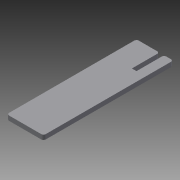
# Autodesk Inventor part: pa28-bellcrank-rigging-tool
Saved by Autodesk Inventor 2015 (Build 190159000, 159)
## iProperties
Created: 2016-01-21
Part Number: pa28-bellcrank-rigging-tool
Material: Generic
Document SubType Name: Modeling
Designer: bovine
Density: 1 g/cm^3
Appearance: Default
Author: bovine
Autodesk Inventor part; units mm, degrees
ref_plane "YZ Plane" through (0, 0, 0) normal (1, 0, 0) x (0, 1, 0)
ref_plane "XZ Plane" through (0, 0, 0) normal (0, 1, 0) x (-1, 0, 0)
ref_plane "XY Plane" through (0, 0, 0) normal (0, 0, 1) x (1, 0, 0)
sketch "Sketch1" plane through (0, 0, 0) normal (0, 1, 0) x (-1, 0, 0)
  line L0 (25.4, 89.6874) -> (0, 89.6874)
  line L1 (0, 89.6874) -> (0, 0)
  line L2 (0, 0) -> (6.35, 0)
  line L3 (25.4, 0) -> (25.4, 89.6874)
  line L4 (9.525, 0) -> (9.525, 19.05)
  line L5 (9.525, 19.05) -> (6.35, 19.05)
  line L6 (6.35, 19.05) -> (6.35, 0)
  line L7 (9.525, 0) -> (25.4, 0)
  dimension "d0" = 25.4
  dimension "d1" = 89.6874
  dimension "d2" = 3.175
  dimension "d3" = 19.05
  constraints: 16 end point, 4 parallel, 1 coincident, 1 horizontal, 1 perpendicular
  measures "d0" distance of L3.start L1.end
  measures "d1" distance of L1.end L0.end
  measures "d2" distance of L5.end L4.end
  measures "d3" distance of L4.end L4.start
extrude "Extrusion1" add sketch "Sketch1" along normal blind 3.175
fillet "Fillet1" radius 1.5748 6 edges at (0, 1.5875, 0) (-25.4, 1.5875, 0) (-6.35, 1.5875, 0) (-9.525, 1.5875, 0) (-25.4, 1.5875, 89.6874) (0, 1.5875, 89.6874)
sketch "Sketch2" plane through (0, 0, 0) normal (0, -1, 0) x (1, 0, 0)
  line L0 (-20.5155, 21.5283) -> (-20.5155, 87.253) construction
  line L1 (-20.5155, 87.253) -> (-16.4672, 87.253) construction
  line L2 (-16.4672, 87.253) -> (-16.4672, 21.5283) construction
  line L3 (-16.4672, 21.5283) -> (-20.5155, 21.5283) construction
  spline S0 degree 2 poles (-19.4608, 23.7637) (-19.2632, 23.7637) (-18.9076, 23.6229) (-18.7841, 23.4969) knots 0 0 0 1 2 2 2
  spline S1 degree 2 poles (-18.7841, 23.4969) (-18.6284, 23.3388) (-18.4679, 22.9115) (-18.4679, 22.5855) knots 0 0 0 1 2 2 2
  line L4 (-18.4679, 22.5855) -> (-18.4679, 22.2422)
  line L5 (-18.4679, 22.2422) -> (-17.3317, 22.2422)
  line L6 (-17.3317, 22.2422) -> (-17.3317, 21.8371)
  line L7 (-17.3317, 21.8371) -> (-20.3797, 21.8371)
  line L8 (-20.3797, 21.8371) -> (-20.3797, 22.6028)
  spline S2 degree 2 poles (-20.3797, 22.6028) (-20.3797, 22.8745) (-20.2908, 23.2549) (-20.1895, 23.4006) knots 0 0 0 1 2 2 2
  spline S3 degree 2 poles (-20.1895, 23.4006) (-20.0734, 23.571) (-19.7152, 23.7637) (-19.4608, 23.7637) knots 0 0 0 1 2 2 2
  spline S4 degree 2 poles (-19.4485, 23.3413) (-19.6066, 23.3413) (-19.8387, 23.2326) (-19.9129, 23.1215) knots 0 0 0 1 2 2 2
  spline S5 degree 2 poles (-19.9129, 23.1215) (-19.9771, 23.0252) (-20.0289, 22.7683) (-20.0289, 22.5781) knots 0 0 0 1 2 2 2
  line L9 (-20.0289, 22.5781) -> (-20.0289, 22.2422)
  line L10 (-20.0289, 22.2422) -> (-18.8137, 22.2422)
  line L11 (-18.8137, 22.2422) -> (-18.8137, 22.5188)
  spline S6 degree 2 poles (-18.8137, 22.5188) (-18.8137, 22.7658) (-18.8927, 23.0696) (-18.9965, 23.1684) knots 0 0 0 1 2 2 2
  spline S7 degree 2 poles (-18.9965, 23.1684) (-19.0879, 23.2598) (-19.3028, 23.3413) (-19.4485, 23.3413) knots 0 0 0 1 2 2 2
  line L12 (-17.3317, 24.5121) -> (-17.3317, 24.1268)
  line L13 (-17.3317, 24.1268) -> (-19.6189, 24.1268)
  line L14 (-19.6189, 24.1268) -> (-19.6189, 24.5121)
  line L15 (-19.6189, 24.5121) -> (-17.3317, 24.5121)
  line L16 (-19.9993, 24.5393) -> (-19.9993, 24.1021)
  line L17 (-19.9993, 24.1021) -> (-20.3994, 24.1021)
  line L18 (-20.3994, 24.1021) -> (-20.3994, 24.5393)
  line L19 (-20.3994, 24.5393) -> (-19.9993, 24.5393)
  spline S8 degree 2 poles (-18.5371, 26.9945) (-17.964, 26.9945) (-17.2872, 26.4486) (-17.2872, 26.0312) knots 0 0 0 1 2 2 2
  spline S9 degree 2 poles (-17.2872, 26.0312) (-17.2872, 25.8607) (-17.3663, 25.5989) (-17.4478, 25.4631) knots 0 0 0 1 2 2 2
  line L20 (-17.4478, 25.4631) -> (-16.4894, 25.4631)
  line L21 (-16.4894, 25.4631) -> (-16.4894, 25.0777)
  line L22 (-16.4894, 25.0777) -> (-19.6189, 25.0777)
  line L23 (-19.6189, 25.0777) -> (-19.6189, 25.4631)
  line L24 (-19.6189, 25.4631) -> (-19.3793, 25.4631)
  spline S10 degree 2 poles (-19.3793, 25.4631) (-19.5102, 25.6063) (-19.6831, 25.9571) (-19.6831, 26.1621) knots 0 0 0 1 2 2 2
  spline S11 degree 2 poles (-19.6831, 26.1621) (-19.6831, 26.5548) (-19.0607, 26.9945) (-18.5371, 26.9945) knots 0 0 0 1 2 2 2
  spline S12 degree 2 poles (-18.4926, 26.5968) (-18.8853, 26.5968) (-19.3176, 26.3473) (-19.3176, 26.0682) knots 0 0 0 1 2 2 2
  spline S13 degree 2 poles (-19.3176, 26.0682) (-19.3176, 25.9052) (-19.1718, 25.5989) (-19.0582, 25.4631) knots 0 0 0 1 2 2 2
  line L25 (-19.0582, 25.4631) -> (-17.759, 25.4631)
  spline S14 degree 2 poles (-17.759, 25.4631) (-17.6874, 25.6137) (-17.633, 25.8286) (-17.633, 25.9669) knots 0 0 0 1 2 2 2
  spline S15 degree 2 poles (-17.633, 25.9669) (-17.633, 26.2658) (-18.0727, 26.5968) (-18.4926, 26.5968) knots 0 0 0 1 2 2 2
  spline S16 degree 2 poles (-17.2798, 28.3876) (-17.2798, 27.8392) (-17.8948, 27.2365) (-18.463, 27.2365) knots 0 0 0 1 2 2 2
  spline S17 degree 2 poles (-18.463, 27.2365) (-19.0212, 27.2365) (-19.6831, 27.8219) (-19.6831, 28.2937) knots 0 0 0 1 2 2 2
  spline S18 degree 2 poles (-19.6831, 28.2937) (-19.6831, 28.5061) (-19.5596, 28.8346) (-19.4287, 28.9557) knots 0 0 0 1 2 2 2
  spline S19 degree 2 poles (-19.4287, 28.9557) (-19.2978, 29.0792) (-18.9199, 29.2101) (-18.6457, 29.2101) knots 0 0 0 1 2 2 2
  line L26 (-18.6457, 29.2101) -> (-18.4358, 29.2101)
  line L27 (-18.4358, 29.2101) -> (-18.4358, 27.6268)
  spline S20 degree 2 poles (-18.4358, 27.6268) (-18.0381, 27.6268) (-17.6157, 28.0269) (-17.6157, 28.3826) knots 0 0 0 1 2 2 2
  spline S21 degree 2 poles (-17.6157, 28.3826) (-17.6157, 28.5086) (-17.6725, 28.7531) (-17.717, 28.8519) knots 0 0 0 1 2 2 2
  spline S22 degree 2 poles (-17.717, 28.8519) (-17.7664, 28.9557) (-17.8529, 29.0989) (-17.8924, 29.1459) knots 0 0 0 1 2 2 2
  line L28 (-17.8924, 29.1459) -> (-17.8924, 29.1681)
  line L29 (-17.8924, 29.1681) -> (-17.4725, 29.1681)
  spline S23 degree 2 poles (-17.4725, 29.1681) (-17.4453, 29.1014) (-17.3663, 28.8989) (-17.344, 28.8198) knots 0 0 0 1 2 2 2
  spline S24 degree 2 poles (-17.344, 28.8198) (-17.3119, 28.7087) (-17.2798, 28.5259) (-17.2798, 28.3876) knots 0 0 0 1 2 2 2
  spline S25 degree 2 poles (-18.7297, 28.8346) (-18.8853, 28.8297) (-19.1126, 28.7655) (-19.1891, 28.7037) knots 0 0 0 1 2 2 2
  spline S26 degree 2 poles (-19.1891, 28.7037) (-19.2756, 28.637) (-19.367, 28.4271) (-19.367, 28.2715) knots 0 0 0 1 2 2 2
  spline S27 degree 2 poles (-19.367, 28.2715) (-19.367, 28.1183) (-19.2756, 27.9034) (-19.1867, 27.8145) knots 0 0 0 1 2 2 2
  spline S28 degree 2 poles (-19.1867, 27.8145) (-19.0953, 27.7281) (-18.8754, 27.6391) (-18.7297, 27.6268) knots 0 0 0 1 2 2 2
  line L30 (-18.7297, 27.6268) -> (-18.7297, 28.8346)
  line L31 (-19.2064, 30.8131) -> (-19.2064, 30.7934)
  spline S29 degree 2 poles (-19.2064, 30.7934) (-19.2188, 30.7489) (-19.2237, 30.6526) (-19.2237, 30.5859) knots 0 0 0 1 2 2 2
  spline S30 degree 2 poles (-19.2237, 30.5859) (-19.2237, 30.4303) (-19.0879, 30.124) (-18.9545, 29.9857) knots 0 0 0 1 2 2 2
  line L32 (-18.9545, 29.9857) -> (-17.3317, 29.9857)
  line L33 (-17.3317, 29.9857) -> (-17.3317, 29.6003)
  line L34 (-17.3317, 29.6003) -> (-19.6189, 29.6003)
  line L35 (-19.6189, 29.6003) -> (-19.6189, 29.9857)
  line L36 (-19.6189, 29.9857) -> (-19.2781, 29.9857)
  spline S31 degree 2 poles (-19.2781, 29.9857) (-19.4658, 30.1956) (-19.6189, 30.5093) (-19.6189, 30.6575) knots 0 0 0 1 2 2 2
  spline S32 degree 2 poles (-19.6189, 30.6575) (-19.6189, 30.7168) (-19.614, 30.7761) (-19.6066, 30.8131) knots 0 0 0 1 2 2 2
  line L37 (-19.6066, 30.8131) -> (-19.2064, 30.8131)
  line L38 (-17.3317, 32.1222) -> (-20.3797, 33.1497)
  line L39 (-20.3797, 33.1497) -> (-20.3797, 33.6487)
  line L40 (-20.3797, 33.6487) -> (-17.3317, 34.6762)
  line L41 (-17.3317, 34.6762) -> (-17.3317, 34.2489)
  line L42 (-17.3317, 34.2489) -> (-18.1838, 33.9723)
  line L43 (-18.1838, 33.9723) -> (-18.1838, 32.8089)
  line L44 (-18.1838, 32.8089) -> (-17.3317, 32.5322)
  line L45 (-17.3317, 32.5322) -> (-17.3317, 32.1222)
  line L46 (-18.5296, 33.8611) -> (-19.9647, 33.3893)
  line L47 (-19.9647, 33.3893) -> (-18.5296, 32.92)
  line L48 (-18.5296, 32.92) -> (-18.5296, 33.8611)
  line L49 (-17.3317, 35.3283) -> (-17.3317, 34.943)
  line L50 (-17.3317, 34.943) -> (-19.6189, 34.943)
  line L51 (-19.6189, 34.943) -> (-19.6189, 35.3283)
  line L52 (-19.6189, 35.3283) -> (-17.3317, 35.3283)
  line L53 (-19.9993, 35.3555) -> (-19.9993, 34.9183)
  line L54 (-19.9993, 34.9183) -> (-20.3994, 34.9183)
  line L55 (-20.3994, 34.9183) -> (-20.3994, 35.3555)
  line L56 (-20.3994, 35.3555) -> (-19.9993, 35.3555)
  line L57 (-17.3317, 36.2867) -> (-17.3317, 35.9013)
  line L58 (-17.3317, 35.9013) -> (-20.5155, 35.9013)
  line L59 (-20.5155, 35.9013) -> (-20.5155, 36.2867)
  line L60 (-20.5155, 36.2867) -> (-17.3317, 36.2867)
  spline S33 degree 2 poles (-17.2798, 37.8452) (-17.2798, 37.2969) (-17.8948, 36.6942) (-18.463, 36.6942) knots 0 0 0 1 2 2 2
  spline S34 degree 2 poles (-18.463, 36.6942) (-19.0212, 36.6942) (-19.6831, 37.2796) (-19.6831, 37.7514) knots 0 0 0 1 2 2 2
  spline S35 degree 2 poles (-19.6831, 37.7514) (-19.6831, 37.9638) (-19.5596, 38.2923) (-19.4287, 38.4134) knots 0 0 0 1 2 2 2
  spline S36 degree 2 poles (-19.4287, 38.4134) (-19.2978, 38.5369) (-18.9199, 38.6678) (-18.6457, 38.6678) knots 0 0 0 1 2 2 2
  line L61 (-18.6457, 38.6678) -> (-18.4358, 38.6678)
  line L62 (-18.4358, 38.6678) -> (-18.4358, 37.0845)
  spline S37 degree 2 poles (-18.4358, 37.0845) (-18.0381, 37.0845) (-17.6157, 37.4846) (-17.6157, 37.8403) knots 0 0 0 1 2 2 2
  spline S38 degree 2 poles (-17.6157, 37.8403) (-17.6157, 37.9663) (-17.6725, 38.2108) (-17.717, 38.3096) knots 0 0 0 1 2 2 2
  spline S39 degree 2 poles (-17.717, 38.3096) (-17.7664, 38.4134) (-17.8529, 38.5566) (-17.8924, 38.6035) knots 0 0 0 1 2 2 2
  line L63 (-17.8924, 38.6035) -> (-17.8924, 38.6258)
  line L64 (-17.8924, 38.6258) -> (-17.4725, 38.6258)
  spline S40 degree 2 poles (-17.4725, 38.6258) (-17.4453, 38.5591) (-17.3663, 38.3565) (-17.344, 38.2775) knots 0 0 0 1 2 2 2
  spline S41 degree 2 poles (-17.344, 38.2775) (-17.3119, 38.1664) (-17.2798, 37.9836) (-17.2798, 37.8452) knots 0 0 0 1 2 2 2
  spline S42 degree 2 poles (-18.7297, 38.2923) (-18.8853, 38.2874) (-19.1126, 38.2232) (-19.1891, 38.1614) knots 0 0 0 1 2 2 2
  spline S43 degree 2 poles (-19.1891, 38.1614) (-19.2756, 38.0947) (-19.367, 37.8848) (-19.367, 37.7292) knots 0 0 0 1 2 2 2
  spline S44 degree 2 poles (-19.367, 37.7292) (-19.367, 37.576) (-19.2756, 37.3611) (-19.1867, 37.2722) knots 0 0 0 1 2 2 2
  spline S45 degree 2 poles (-19.1867, 37.2722) (-19.0953, 37.1858) (-18.8754, 37.0968) (-18.7297, 37.0845) knots 0 0 0 1 2 2 2
  line L65 (-18.7297, 37.0845) -> (-18.7297, 38.2923)
  line L66 (-19.2064, 40.2708) -> (-19.2064, 40.251)
  spline S46 degree 2 poles (-19.2064, 40.251) (-19.2188, 40.2066) (-19.2237, 40.1103) (-19.2237, 40.0436) knots 0 0 0 1 2 2 2
  spline S47 degree 2 poles (-19.2237, 40.0436) (-19.2237, 39.888) (-19.0879, 39.5817) (-18.9545, 39.4433) knots 0 0 0 1 2 2 2
  line L67 (-18.9545, 39.4433) -> (-17.3317, 39.4433)
  line L68 (-17.3317, 39.4433) -> (-17.3317, 39.058)
  line L69 (-17.3317, 39.058) -> (-19.6189, 39.058)
  line L70 (-19.6189, 39.058) -> (-19.6189, 39.4433)
  line L71 (-19.6189, 39.4433) -> (-19.2781, 39.4433)
  spline S48 degree 2 poles (-19.2781, 39.4433) (-19.4658, 39.6533) (-19.6189, 39.967) (-19.6189, 40.1152) knots 0 0 0 1 2 2 2
  spline S49 degree 2 poles (-19.6189, 40.1152) (-19.6189, 40.1745) (-19.614, 40.2338) (-19.6066, 40.2708) knots 0 0 0 1 2 2 2
  line L72 (-19.6066, 40.2708) -> (-19.2064, 40.2708)
  spline S50 degree 2 poles (-18.4753, 42.4494) (-17.8973, 42.4494) (-17.2675, 41.8936) (-17.2675, 41.4292) knots 0 0 0 1 2 2 2
  spline S51 degree 2 poles (-17.2675, 41.4292) (-17.2675, 40.9525) (-17.9171, 40.4067) (-18.4753, 40.4067) knots 0 0 0 1 2 2 2
  spline S52 degree 2 poles (-18.4753, 40.4067) (-19.0483, 40.4067) (-19.6831, 40.9698) (-19.6831, 41.4292) knots 0 0 0 1 2 2 2
  spline S53 degree 2 poles (-19.6831, 41.4292) (-19.6831, 41.8936) (-19.0508, 42.4494) (-18.4753, 42.4494) knots 0 0 0 1 2 2 2
  spline S54 degree 2 poles (-18.4753, 42.0517) (-18.9199, 42.0517) (-19.3522, 41.7281) (-19.3522, 41.4292) knots 0 0 0 1 2 2 2
  spline S55 degree 2 poles (-19.3522, 41.4292) (-19.3522, 41.1304) (-18.9199, 40.8043) (-18.4753, 40.8043) knots 0 0 0 1 2 2 2
  spline S56 degree 2 poles (-18.4753, 40.8043) (-18.043, 40.8043) (-17.5984, 41.1304) (-17.5984, 41.4292) knots 0 0 0 1 2 2 2
  spline S57 degree 2 poles (-17.5984, 41.4292) (-17.5984, 41.7256) (-18.0356, 42.0517) (-18.4753, 42.0517) knots 0 0 0 1 2 2 2
  line L73 (-17.3317, 44.6403) -> (-17.3317, 44.2549)
  line L74 (-17.3317, 44.2549) -> (-18.6359, 44.2549)
  spline S58 degree 2 poles (-18.6359, 44.2549) (-18.7939, 44.2549) (-19.0656, 44.2253) (-19.1471, 44.1808) knots 0 0 0 1 2 2 2
  spline S59 degree 2 poles (-19.1471, 44.1808) (-19.2336, 44.1339) (-19.3176, 43.9659) (-19.3176, 43.8227) knots 0 0 0 1 2 2 2
  spline S60 degree 2 poles (-19.3176, 43.8227) (-19.3176, 43.6794) (-19.1644, 43.3756) (-19.0409, 43.2299) knots 0 0 0 1 2 2 2
  line L75 (-19.0409, 43.2299) -> (-17.3317, 43.2299)
  line L76 (-17.3317, 43.2299) -> (-17.3317, 42.8446)
  line L77 (-17.3317, 42.8446) -> (-19.6189, 42.8446)
  line L78 (-19.6189, 42.8446) -> (-19.6189, 43.2299)
  line L79 (-19.6189, 43.2299) -> (-19.3645, 43.2299)
  spline S61 degree 2 poles (-19.3645, 43.2299) (-19.5201, 43.4028) (-19.6831, 43.7362) (-19.6831, 43.924) knots 0 0 0 1 2 2 2
  spline S62 degree 2 poles (-19.6831, 43.924) (-19.6831, 44.2599) (-19.2385, 44.6403) (-18.8162, 44.6403) knots 0 0 0 1 2 2 2
  line L80 (-18.8162, 44.6403) -> (-17.3317, 44.6403)
  spline S63 degree 2 poles (-18.2678, 48.5873) (-18.0406, 48.5873) (-17.6923, 48.4144) (-17.5787, 48.2712) knots 0 0 0 1 2 2 2
  spline S64 degree 2 poles (-17.5787, 48.2712) (-17.4453, 48.0983) (-17.3317, 47.7056) (-17.3317, 47.3943) knots 0 0 0 1 2 2 2
  line L81 (-17.3317, 47.3943) -> (-17.3317, 46.5199)
  line L82 (-17.3317, 46.5199) -> (-20.3797, 46.5199)
  line L83 (-20.3797, 46.5199) -> (-20.3797, 47.3276)
  spline S65 degree 2 poles (-20.3797, 47.3276) (-20.3797, 47.6537) (-20.3377, 47.9797) (-20.2562, 48.1279) knots 0 0 0 1 2 2 2
  spline S66 degree 2 poles (-20.2562, 48.1279) (-20.1697, 48.2934) (-19.8857, 48.4441) (-19.693, 48.4441) knots 0 0 0 1 2 2 2
  spline S67 degree 2 poles (-19.693, 48.4441) (-19.4781, 48.4441) (-19.1373, 48.2168) (-19.0409, 48.0168) knots 0 0 0 1 2 2 2
  line L84 (-19.0409, 48.0168) -> (-19.0261, 48.0168)
  spline S68 degree 2 poles (-19.0261, 48.0168) (-18.952, 48.2885) (-18.5593, 48.5873) (-18.2678, 48.5873) knots 0 0 0 1 2 2 2
  spline S69 degree 2 poles (-18.2505, 48.165) (-18.4234, 48.165) (-18.6457, 48.0662) (-18.7248, 47.918) knots 0 0 0 1 2 2 2
  spline S70 degree 2 poles (-18.7248, 47.918) (-18.7742, 47.8216) (-18.8038, 47.5944) (-18.8038, 47.3845) knots 0 0 0 1 2 2 2
  line L85 (-18.8038, 47.3845) -> (-18.8038, 46.925)
  line L86 (-18.8038, 46.925) -> (-17.6775, 46.925)
  line L87 (-17.6775, 46.925) -> (-17.6775, 47.2535)
  spline S71 degree 2 poles (-17.6775, 47.2535) (-17.6775, 47.5203) (-17.7269, 47.8266) (-17.8059, 47.9451) knots 0 0 0 1 2 2 2
  spline S72 degree 2 poles (-17.8059, 47.9451) (-17.8874, 48.0588) (-18.09, 48.165) (-18.2505, 48.165) knots 0 0 0 1 2 2 2
  spline S73 degree 2 poles (-19.6362, 48.0217) (-19.7449, 48.0217) (-19.9079, 47.9476) (-19.9548, 47.8661) knots 0 0 0 1 2 2 2
  spline S74 degree 2 poles (-19.9548, 47.8661) (-20.0092, 47.7673) (-20.0339, 47.5277) (-20.0339, 47.3128) knots 0 0 0 1 2 2 2
  line L88 (-20.0339, 47.3128) -> (-20.0339, 46.925)
  line L89 (-20.0339, 46.925) -> (-19.1422, 46.925)
  line L90 (-19.1422, 46.925) -> (-19.1422, 47.3845)
  spline S75 degree 2 poles (-19.1422, 47.3845) (-19.1422, 47.5746) (-19.1817, 47.755) (-19.2435, 47.8513) knots 0 0 0 1 2 2 2
  spline S76 degree 2 poles (-19.2435, 47.8513) (-19.3028, 47.9451) (-19.4929, 48.0217) (-19.6362, 48.0217) knots 0 0 0 1 2 2 2
  spline S77 degree 2 poles (-17.2798, 49.9533) (-17.2798, 49.4049) (-17.8948, 48.8022) (-18.463, 48.8022) knots 0 0 0 1 2 2 2
  spline S78 degree 2 poles (-18.463, 48.8022) (-19.0212, 48.8022) (-19.6831, 49.3876) (-19.6831, 49.8594) knots 0 0 0 1 2 2 2
  spline S79 degree 2 poles (-19.6831, 49.8594) (-19.6831, 50.0718) (-19.5596, 50.4003) (-19.4287, 50.5214) knots 0 0 0 1 2 2 2
  spline S80 degree 2 poles (-19.4287, 50.5214) (-19.2978, 50.6449) (-18.9199, 50.7758) (-18.6457, 50.7758) knots 0 0 0 1 2 2 2
  line L91 (-18.6457, 50.7758) -> (-18.4358, 50.7758)
  line L92 (-18.4358, 50.7758) -> (-18.4358, 49.1925)
  spline S81 degree 2 poles (-18.4358, 49.1925) (-18.0381, 49.1925) (-17.6157, 49.5926) (-17.6157, 49.9483) knots 0 0 0 1 2 2 2
  spline S82 degree 2 poles (-17.6157, 49.9483) (-17.6157, 50.0743) (-17.6725, 50.3188) (-17.717, 50.4176) knots 0 0 0 1 2 2 2
  spline S83 degree 2 poles (-17.717, 50.4176) (-17.7664, 50.5214) (-17.8529, 50.6646) (-17.8924, 50.7116) knots 0 0 0 1 2 2 2
  line L93 (-17.8924, 50.7116) -> (-17.8924, 50.7338)
  line L94 (-17.8924, 50.7338) -> (-17.4725, 50.7338)
  spline S84 degree 2 poles (-17.4725, 50.7338) (-17.4453, 50.6671) (-17.3663, 50.4646) (-17.344, 50.3855) knots 0 0 0 1 2 2 2
  spline S85 degree 2 poles (-17.344, 50.3855) (-17.3119, 50.2744) (-17.2798, 50.0916) (-17.2798, 49.9533) knots 0 0 0 1 2 2 2
  spline S86 degree 2 poles (-18.7297, 50.4003) (-18.8853, 50.3954) (-19.1126, 50.3312) (-19.1891, 50.2694) knots 0 0 0 1 2 2 2
  spline S87 degree 2 poles (-19.1891, 50.2694) (-19.2756, 50.2027) (-19.367, 49.9928) (-19.367, 49.8372) knots 0 0 0 1 2 2 2
  spline S88 degree 2 poles (-19.367, 49.8372) (-19.367, 49.684) (-19.2756, 49.4691) (-19.1867, 49.3802) knots 0 0 0 1 2 2 2
  spline S89 degree 2 poles (-19.1867, 49.3802) (-19.0953, 49.2938) (-18.8754, 49.2049) (-18.7297, 49.1925) knots 0 0 0 1 2 2 2
  line L95 (-18.7297, 49.1925) -> (-18.7297, 50.4003)
  line L96 (-17.3317, 51.5588) -> (-17.3317, 51.1735)
  line L97 (-17.3317, 51.1735) -> (-20.5155, 51.1735)
  line L98 (-20.5155, 51.1735) -> (-20.5155, 51.5588)
  line L99 (-20.5155, 51.5588) -> (-17.3317, 51.5588)
  line L100 (-17.3317, 52.5171) -> (-17.3317, 52.1318)
  line L101 (-17.3317, 52.1318) -> (-20.5155, 52.1318)
  line L102 (-20.5155, 52.1318) -> (-20.5155, 52.5171)
  line L103 (-20.5155, 52.5171) -> (-17.3317, 52.5171)
  spline S90 degree 2 poles (-17.2798, 53.9917) (-17.2798, 53.7546) (-17.4255, 53.3619) (-17.5737, 53.2211) knots 0 0 0 1 2 2 2
  spline S91 degree 2 poles (-17.5737, 53.2211) (-17.7195, 53.0803) (-18.169, 52.9247) (-18.4704, 52.9247) knots 0 0 0 1 2 2 2
  spline S92 degree 2 poles (-18.4704, 52.9247) (-18.7717, 52.9247) (-19.2114, 53.0852) (-19.3596, 53.2211) knots 0 0 0 1 2 2 2
  spline S93 degree 2 poles (-19.3596, 53.2211) (-19.5102, 53.357) (-19.6708, 53.7596) (-19.6708, 53.9917) knots 0 0 0 1 2 2 2
  spline S94 degree 2 poles (-19.6708, 53.9917) (-19.6708, 54.1795) (-19.5646, 54.5302) (-19.4954, 54.6661) knots 0 0 0 1 2 2 2
  line L104 (-19.4954, 54.6661) -> (-19.0632, 54.6661)
  line L105 (-19.0632, 54.6661) -> (-19.0632, 54.6438)
  spline S95 degree 2 poles (-19.0632, 54.6438) (-19.0977, 54.6018) (-19.1867, 54.4734) (-19.2336, 54.382) knots 0 0 0 1 2 2 2
  spline S96 degree 2 poles (-19.2336, 54.382) (-19.2731, 54.3005) (-19.3349, 54.0831) (-19.3349, 53.9843) knots 0 0 0 1 2 2 2
  spline S97 degree 2 poles (-19.3349, 53.9843) (-19.3349, 53.6855) (-18.8829, 53.3224) (-18.4704, 53.3224) knots 0 0 0 1 2 2 2
  spline S98 degree 2 poles (-18.4704, 53.3224) (-18.0677, 53.3224) (-17.6157, 53.6731) (-17.6157, 53.9843) knots 0 0 0 1 2 2 2
  spline S99 degree 2 poles (-17.6157, 53.9843) (-17.6157, 54.1721) (-17.7713, 54.5129) (-17.8924, 54.6438) knots 0 0 0 1 2 2 2
  line L106 (-17.8924, 54.6438) -> (-17.8924, 54.6661)
  line L107 (-17.8924, 54.6661) -> (-17.4601, 54.6661)
  spline S100 degree 2 poles (-17.4601, 54.6661) (-17.433, 54.6092) (-17.3564, 54.4363) (-17.3391, 54.3672) knots 0 0 0 1 2 2 2
  spline S101 degree 2 poles (-17.3391, 54.3672) (-17.3095, 54.2684) (-17.2798, 54.1128) (-17.2798, 53.9917) knots 0 0 0 1 2 2 2
  line L108 (-19.2064, 56.2296) -> (-19.2064, 56.2098)
  spline S102 degree 2 poles (-19.2064, 56.2098) (-19.2188, 56.1654) (-19.2237, 56.069) (-19.2237, 56.0023) knots 0 0 0 1 2 2 2
  spline S103 degree 2 poles (-19.2237, 56.0023) (-19.2237, 55.8467) (-19.0879, 55.5404) (-18.9545, 55.4021) knots 0 0 0 1 2 2 2
  line L109 (-18.9545, 55.4021) -> (-17.3317, 55.4021)
  line L110 (-17.3317, 55.4021) -> (-17.3317, 55.0168)
  line L111 (-17.3317, 55.0168) -> (-19.6189, 55.0168)
  line L112 (-19.6189, 55.0168) -> (-19.6189, 55.4021)
  line L113 (-19.6189, 55.4021) -> (-19.2781, 55.4021)
  spline S104 degree 2 poles (-19.2781, 55.4021) (-19.4658, 55.6121) (-19.6189, 55.9258) (-19.6189, 56.074) knots 0 0 0 1 2 2 2
  spline S105 degree 2 poles (-19.6189, 56.074) (-19.6189, 56.1332) (-19.614, 56.1925) (-19.6066, 56.2296) knots 0 0 0 1 2 2 2
  line L114 (-19.6066, 56.2296) -> (-19.2064, 56.2296)
  spline S106 degree 2 poles (-17.5737, 57.803) (-17.5392, 57.7561) (-17.4157, 57.598) (-17.3786, 57.5239) knots 0 0 0 1 2 2 2
  spline S107 degree 2 poles (-17.3786, 57.5239) (-17.3243, 57.4226) (-17.2675, 57.2324) (-17.2675, 57.0595) knots 0 0 0 1 2 2 2
  spline S108 degree 2 poles (-17.2675, 57.0595) (-17.2675, 56.9187) (-17.3737, 56.6643) (-17.47, 56.568) knots 0 0 0 1 2 2 2
  spline S109 degree 2 poles (-17.47, 56.568) (-17.5639, 56.4766) (-17.8405, 56.3654) (-17.9936, 56.3654) knots 0 0 0 1 2 2 2
  spline S110 degree 2 poles (-17.9936, 56.3654) (-18.2308, 56.3654) (-18.5667, 56.5655) (-18.663, 56.7829) knots 0 0 0 1 2 2 2
  spline S111 degree 2 poles (-18.663, 56.7829) (-18.7519, 56.9755) (-18.8186, 57.4992) (-18.8359, 57.803) knots 0 0 0 1 2 2 2
  line L115 (-18.8359, 57.803) -> (-18.91, 57.803)
  spline S112 degree 2 poles (-18.91, 57.803) (-19.0434, 57.803) (-19.2089, 57.7215) (-19.2558, 57.6474) knots 0 0 0 1 2 2 2
  spline S113 degree 2 poles (-19.2558, 57.6474) (-19.3028, 57.5733) (-19.3324, 57.3608) (-19.3324, 57.2472) knots 0 0 0 1 2 2 2
  spline S114 degree 2 poles (-19.3324, 57.2472) (-19.3324, 57.1138) (-19.2534, 56.7532) (-19.1768, 56.5729) knots 0 0 0 1 2 2 2
  line L116 (-19.1768, 56.5729) -> (-19.1768, 56.5507)
  line L117 (-19.1768, 56.5507) -> (-19.5695, 56.5507)
  spline S115 degree 2 poles (-19.5695, 56.5507) (-19.5992, 56.6569) (-19.6733, 57.0546) (-19.6733, 57.2497) knots 0 0 0 1 2 2 2
  spline S116 degree 2 poles (-19.6733, 57.2497) (-19.6733, 57.4868) (-19.5992, 57.8104) (-19.5028, 57.9388) knots 0 0 0 1 2 2 2
  spline S117 degree 2 poles (-19.5028, 57.9388) (-19.409, 58.0648) (-19.1101, 58.1883) (-18.8952, 58.1883) knots 0 0 0 1 2 2 2
  line L118 (-18.8952, 58.1883) -> (-17.3317, 58.1883)
  line L119 (-17.3317, 58.1883) -> (-17.3317, 57.803)
  line L120 (-17.3317, 57.803) -> (-17.5737, 57.803)
  line L121 (-17.8948, 57.803) -> (-18.5296, 57.803)
  spline S118 degree 2 poles (-18.5296, 57.803) (-18.5173, 57.6647) (-18.4753, 57.2472) (-18.4358, 57.1163) knots 0 0 0 1 2 2 2
  spline S119 degree 2 poles (-18.4358, 57.1163) (-18.3889, 56.9632) (-18.1937, 56.7631) (-18.0208, 56.7631) knots 0 0 0 1 2 2 2
  spline S120 degree 2 poles (-18.0208, 56.7631) (-17.8232, 56.7631) (-17.6231, 56.9854) (-17.6231, 57.1978) knots 0 0 0 1 2 2 2
  spline S121 degree 2 poles (-17.6231, 57.1978) (-17.6231, 57.3781) (-17.7788, 57.6745) (-17.8948, 57.803) knots 0 0 0 1 2 2 2
  line L122 (-17.3317, 60.5249) -> (-17.3317, 60.1396)
  line L123 (-17.3317, 60.1396) -> (-18.6359, 60.1396)
  spline S122 degree 2 poles (-18.6359, 60.1396) (-18.7939, 60.1396) (-19.0656, 60.11) (-19.1471, 60.0655) knots 0 0 0 1 2 2 2
  spline S123 degree 2 poles (-19.1471, 60.0655) (-19.2336, 60.0186) (-19.3176, 59.8506) (-19.3176, 59.7074) knots 0 0 0 1 2 2 2
  spline S124 degree 2 poles (-19.3176, 59.7074) (-19.3176, 59.5641) (-19.1644, 59.2603) (-19.0409, 59.1146) knots 0 0 0 1 2 2 2
  line L124 (-19.0409, 59.1146) -> (-17.3317, 59.1146)
  line L125 (-17.3317, 59.1146) -> (-17.3317, 58.7292)
  line L126 (-17.3317, 58.7292) -> (-19.6189, 58.7292)
  line L127 (-19.6189, 58.7292) -> (-19.6189, 59.1146)
  line L128 (-19.6189, 59.1146) -> (-19.3645, 59.1146)
  spline S125 degree 2 poles (-19.3645, 59.1146) (-19.5201, 59.2875) (-19.6831, 59.6209) (-19.6831, 59.8086) knots 0 0 0 1 2 2 2
  spline S126 degree 2 poles (-19.6831, 59.8086) (-19.6831, 60.1446) (-19.2385, 60.5249) (-18.8162, 60.5249) knots 0 0 0 1 2 2 2
  line L129 (-18.8162, 60.5249) -> (-17.3317, 60.5249)
  line L130 (-17.3317, 62.9604) -> (-17.3317, 62.454)
  line L131 (-17.3317, 62.454) -> (-18.4358, 61.6043)
  line L132 (-18.4358, 61.6043) -> (-18.2876, 61.4512)
  line L133 (-18.2876, 61.4512) -> (-17.3317, 61.4512)
  line L134 (-17.3317, 61.4512) -> (-17.3317, 61.0659)
  line L135 (-17.3317, 61.0659) -> (-20.5155, 61.0659)
  line L136 (-20.5155, 61.0659) -> (-20.5155, 61.4512)
  line L137 (-20.5155, 61.4512) -> (-18.6531, 61.4512)
  line L138 (-18.6531, 61.4512) -> (-19.6189, 62.3552)
  line L139 (-19.6189, 62.3552) -> (-19.6189, 62.8344)
  line L140 (-19.6189, 62.8344) -> (-18.663, 61.8958)
  line L141 (-18.663, 61.8958) -> (-17.3317, 62.9604)
  line L142 (-17.3317, 66.8506) -> (-17.3317, 66.3245)
  line L143 (-17.3317, 66.3245) -> (-18.5445, 65.3612)
  line L144 (-18.5445, 65.3612) -> (-18.5445, 64.8969)
  line L145 (-18.5445, 64.8969) -> (-17.3317, 64.8969)
  line L146 (-17.3317, 64.8969) -> (-17.3317, 64.4918)
  line L147 (-17.3317, 64.4918) -> (-20.3797, 64.4918)
  line L148 (-20.3797, 64.4918) -> (-20.3797, 65.2772)
  spline S127 degree 2 poles (-20.3797, 65.2772) (-20.3797, 65.5391) (-20.3229, 65.8923) (-20.2191, 66.0528) knots 0 0 0 1 2 2 2
  spline S128 degree 2 poles (-20.2191, 66.0528) (-20.1154, 66.2134) (-19.7918, 66.3986) (-19.5522, 66.3986) knots 0 0 0 1 2 2 2
  spline S129 degree 2 poles (-19.5522, 66.3986) (-19.2188, 66.3986) (-18.7668, 66.0578) (-18.6581, 65.7663) knots 0 0 0 1 2 2 2
  line L149 (-18.6581, 65.7663) -> (-17.3317, 66.8506)
  spline S130 degree 2 poles (-19.5201, 65.9763) (-19.6535, 65.9763) (-19.8585, 65.8824) (-19.9252, 65.7836) knots 0 0 0 1 2 2 2
  spline S131 degree 2 poles (-19.9252, 65.7836) (-19.982, 65.6972) (-20.0289, 65.4674) (-20.0289, 65.2995) knots 0 0 0 1 2 2 2
  line L150 (-20.0289, 65.2995) -> (-20.0289, 64.8969)
  line L151 (-20.0289, 64.8969) -> (-18.8829, 64.8969)
  line L152 (-18.8829, 64.8969) -> (-18.8829, 65.2525)
  spline S132 degree 2 poles (-18.8829, 65.2525) (-18.8829, 65.4279) (-18.9446, 65.707) (-19.0409, 65.8034) knots 0 0 0 1 2 2 2
  spline S133 degree 2 poles (-19.0409, 65.8034) (-19.1249, 65.8923) (-19.362, 65.9763) (-19.5201, 65.9763) knots 0 0 0 1 2 2 2
  line L153 (-17.3317, 67.4558) -> (-17.3317, 67.0705)
  line L154 (-17.3317, 67.0705) -> (-19.6189, 67.0705)
  line L155 (-19.6189, 67.0705) -> (-19.6189, 67.4558)
  line L156 (-19.6189, 67.4558) -> (-17.3317, 67.4558)
  line L157 (-19.9993, 67.483) -> (-19.9993, 67.0458)
  line L158 (-19.9993, 67.0458) -> (-20.3994, 67.0458)
  line L159 (-20.3994, 67.0458) -> (-20.3994, 67.483)
  line L160 (-20.3994, 67.483) -> (-19.9993, 67.483)
  spline S134 degree 2 poles (-16.9661, 68.1029) (-16.9488, 68.1425) (-16.8945, 68.2931) (-16.8723, 68.3895) knots 0 0 0 1 2 2 2
  spline S135 degree 2 poles (-16.8723, 68.3895) (-16.8451, 68.4957) (-16.813, 68.676) (-16.813, 68.7822) knots 0 0 0 1 2 2 2
  spline S136 degree 2 poles (-16.813, 68.7822) (-16.813, 68.96) (-16.9068, 69.207) (-16.9908, 69.2762) knots 0 0 0 1 2 2 2
  spline S137 degree 2 poles (-16.9908, 69.2762) (-17.0748, 69.3429) (-17.2946, 69.3948) (-17.4354, 69.3948) knots 0 0 0 1 2 2 2
  line L161 (-17.4354, 69.3948) -> (-17.6355, 69.3948)
  spline S138 degree 2 poles (-17.6355, 69.3948) (-17.4996, 69.2392) (-17.3712, 68.9403) (-17.3712, 68.7155) knots 0 0 0 1 2 2 2
  spline S139 degree 2 poles (-17.3712, 68.7155) (-17.3712, 68.3252) (-17.9517, 67.8634) (-18.4975, 67.8634) knots 0 0 0 1 2 2 2
  spline S140 degree 2 poles (-18.4975, 67.8634) (-18.7816, 67.8634) (-19.2212, 68.0239) (-19.3769, 68.1573) knots 0 0 0 1 2 2 2
  spline S141 degree 2 poles (-19.3769, 68.1573) (-19.5226, 68.2857) (-19.6831, 68.6389) (-19.6831, 68.8267) knots 0 0 0 1 2 2 2
  spline S142 degree 2 poles (-19.6831, 68.8267) (-19.6831, 69.0045) (-19.5992, 69.2639) (-19.5226, 69.3948) knots 0 0 0 1 2 2 2
  line L162 (-19.5226, 69.3948) -> (-19.6189, 69.417)
  line L163 (-19.6189, 69.417) -> (-19.6189, 69.7801)
  line L164 (-19.6189, 69.7801) -> (-17.5935, 69.7801)
  spline S143 degree 2 poles (-17.5935, 69.7801) (-17.0106, 69.7801) (-16.4672, 69.2737) (-16.4672, 68.7526) knots 0 0 0 1 2 2 2
  spline S144 degree 2 poles (-16.4672, 68.7526) (-16.4672, 68.5846) (-16.5215, 68.2339) (-16.566, 68.0832) knots 0 0 0 1 2 2 2
  line L165 (-16.566, 68.0832) -> (-16.9661, 68.0832)
  line L166 (-16.9661, 68.0832) -> (-16.9661, 68.1029)
  line L167 (-17.9517, 69.3948) -> (-19.2089, 69.3948)
  spline S145 degree 2 poles (-19.2089, 69.3948) (-19.2781, 69.2515) (-19.3373, 69.0094) (-19.3373, 68.8884) knots 0 0 0 1 2 2 2
  spline S146 degree 2 poles (-19.3373, 68.8884) (-19.3373, 68.597) (-18.9076, 68.261) (-18.5049, 68.261) knots 0 0 0 1 2 2 2
  spline S147 degree 2 poles (-18.5049, 68.261) (-18.1246, 68.261) (-17.7269, 68.5154) (-17.7269, 68.802) knots 0 0 0 1 2 2 2
  spline S148 degree 2 poles (-17.7269, 68.802) (-17.7269, 68.9526) (-17.8454, 69.2688) (-17.9517, 69.3948) knots 0 0 0 1 2 2 2
  spline S149 degree 2 poles (-16.9661, 70.4198) (-16.9488, 70.4593) (-16.8945, 70.61) (-16.8723, 70.7063) knots 0 0 0 1 2 2 2
  spline S150 degree 2 poles (-16.8723, 70.7063) (-16.8451, 70.8126) (-16.813, 70.9929) (-16.813, 71.0991) knots 0 0 0 1 2 2 2
  spline S151 degree 2 poles (-16.813, 71.0991) (-16.813, 71.2769) (-16.9068, 71.5239) (-16.9908, 71.5931) knots 0 0 0 1 2 2 2
  spline S152 degree 2 poles (-16.9908, 71.5931) (-17.0748, 71.6598) (-17.2946, 71.7116) (-17.4354, 71.7116) knots 0 0 0 1 2 2 2
  line L168 (-17.4354, 71.7116) -> (-17.6355, 71.7116)
  spline S153 degree 2 poles (-17.6355, 71.7116) (-17.4996, 71.556) (-17.3712, 71.2572) (-17.3712, 71.0324) knots 0 0 0 1 2 2 2
  spline S154 degree 2 poles (-17.3712, 71.0324) (-17.3712, 70.6421) (-17.9517, 70.1802) (-18.4975, 70.1802) knots 0 0 0 1 2 2 2
  spline S155 degree 2 poles (-18.4975, 70.1802) (-18.7816, 70.1802) (-19.2212, 70.3408) (-19.3769, 70.4742) knots 0 0 0 1 2 2 2
  spline S156 degree 2 poles (-19.3769, 70.4742) (-19.5226, 70.6026) (-19.6831, 70.9558) (-19.6831, 71.1435) knots 0 0 0 1 2 2 2
  spline S157 degree 2 poles (-19.6831, 71.1435) (-19.6831, 71.3214) (-19.5992, 71.5807) (-19.5226, 71.7116) knots 0 0 0 1 2 2 2
  line L169 (-19.5226, 71.7116) -> (-19.6189, 71.7339)
  line L170 (-19.6189, 71.7339) -> (-19.6189, 72.097)
  line L171 (-19.6189, 72.097) -> (-17.5935, 72.097)
  spline S158 degree 2 poles (-17.5935, 72.097) (-17.0106, 72.097) (-16.4672, 71.5906) (-16.4672, 71.0694) knots 0 0 0 1 2 2 2
  spline S159 degree 2 poles (-16.4672, 71.0694) (-16.4672, 70.9015) (-16.5215, 70.5507) (-16.566, 70.4001) knots 0 0 0 1 2 2 2
  line L172 (-16.566, 70.4001) -> (-16.9661, 70.4001)
  line L173 (-16.9661, 70.4001) -> (-16.9661, 70.4198)
  line L174 (-17.9517, 71.7116) -> (-19.2089, 71.7116)
  spline S160 degree 2 poles (-19.2089, 71.7116) (-19.2781, 71.5684) (-19.3373, 71.3263) (-19.3373, 71.2053) knots 0 0 0 1 2 2 2
  spline S161 degree 2 poles (-19.3373, 71.2053) (-19.3373, 70.9138) (-18.9076, 70.5779) (-18.5049, 70.5779) knots 0 0 0 1 2 2 2
  spline S162 degree 2 poles (-18.5049, 70.5779) (-18.1246, 70.5779) (-17.7269, 70.8323) (-17.7269, 71.1188) knots 0 0 0 1 2 2 2
  spline S163 degree 2 poles (-17.7269, 71.1188) (-17.7269, 71.2695) (-17.8454, 71.5857) (-17.9517, 71.7116) knots 0 0 0 1 2 2 2
  line L175 (-17.3317, 73.0479) -> (-17.3317, 72.6626)
  line L176 (-17.3317, 72.6626) -> (-19.6189, 72.6626)
  line L177 (-19.6189, 72.6626) -> (-19.6189, 73.0479)
  line L178 (-19.6189, 73.0479) -> (-17.3317, 73.0479)
  line L179 (-19.9993, 73.0751) -> (-19.9993, 72.6379)
  line L180 (-19.9993, 72.6379) -> (-20.3994, 72.6379)
  line L181 (-20.3994, 72.6379) -> (-20.3994, 73.0751)
  line L182 (-20.3994, 73.0751) -> (-19.9993, 73.0751)
  line L183 (-17.3317, 75.4093) -> (-17.3317, 75.0239)
  line L184 (-17.3317, 75.0239) -> (-18.6359, 75.0239)
  spline S164 degree 2 poles (-18.6359, 75.0239) (-18.7939, 75.0239) (-19.0656, 74.9943) (-19.1471, 74.9498) knots 0 0 0 1 2 2 2
  spline S165 degree 2 poles (-19.1471, 74.9498) (-19.2336, 74.9029) (-19.3176, 74.7349) (-19.3176, 74.5917) knots 0 0 0 1 2 2 2
  spline S166 degree 2 poles (-19.3176, 74.5917) (-19.3176, 74.4484) (-19.1644, 74.1446) (-19.0409, 73.9989) knots 0 0 0 1 2 2 2
  line L185 (-19.0409, 73.9989) -> (-17.3317, 73.9989)
  line L186 (-17.3317, 73.9989) -> (-17.3317, 73.6136)
  line L187 (-17.3317, 73.6136) -> (-19.6189, 73.6136)
  line L188 (-19.6189, 73.6136) -> (-19.6189, 73.9989)
  line L189 (-19.6189, 73.9989) -> (-19.3645, 73.9989)
  spline S167 degree 2 poles (-19.3645, 73.9989) (-19.5201, 74.1718) (-19.6831, 74.5052) (-19.6831, 74.693) knots 0 0 0 1 2 2 2
  spline S168 degree 2 poles (-19.6831, 74.693) (-19.6831, 75.0289) (-19.2385, 75.4093) (-18.8162, 75.4093) knots 0 0 0 1 2 2 2
  line L190 (-18.8162, 75.4093) -> (-17.3317, 75.4093)
  spline S169 degree 2 poles (-16.9661, 76.0317) (-16.9488, 76.0712) (-16.8945, 76.2219) (-16.8723, 76.3182) knots 0 0 0 1 2 2 2
  spline S170 degree 2 poles (-16.8723, 76.3182) (-16.8451, 76.4244) (-16.813, 76.6047) (-16.813, 76.711) knots 0 0 0 1 2 2 2
  spline S171 degree 2 poles (-16.813, 76.711) (-16.813, 76.8888) (-16.9068, 77.1358) (-16.9908, 77.205) knots 0 0 0 1 2 2 2
  spline S172 degree 2 poles (-16.9908, 77.205) (-17.0748, 77.2716) (-17.2946, 77.3235) (-17.4354, 77.3235) knots 0 0 0 1 2 2 2
  line L191 (-17.4354, 77.3235) -> (-17.6355, 77.3235)
  spline S173 degree 2 poles (-17.6355, 77.3235) (-17.4996, 77.1679) (-17.3712, 76.869) (-17.3712, 76.6443) knots 0 0 0 1 2 2 2
  spline S174 degree 2 poles (-17.3712, 76.6443) (-17.3712, 76.254) (-17.9517, 75.7921) (-18.4975, 75.7921) knots 0 0 0 1 2 2 2
  spline S175 degree 2 poles (-18.4975, 75.7921) (-18.7816, 75.7921) (-19.2212, 75.9527) (-19.3769, 76.086) knots 0 0 0 1 2 2 2
  spline S176 degree 2 poles (-19.3769, 76.086) (-19.5226, 76.2145) (-19.6831, 76.5677) (-19.6831, 76.7554) knots 0 0 0 1 2 2 2
  spline S177 degree 2 poles (-19.6831, 76.7554) (-19.6831, 76.9333) (-19.5992, 77.1926) (-19.5226, 77.3235) knots 0 0 0 1 2 2 2
  line L192 (-19.5226, 77.3235) -> (-19.6189, 77.3457)
  line L193 (-19.6189, 77.3457) -> (-19.6189, 77.7088)
  line L194 (-19.6189, 77.7088) -> (-17.5935, 77.7088)
  spline S178 degree 2 poles (-17.5935, 77.7088) (-17.0106, 77.7088) (-16.4672, 77.2025) (-16.4672, 76.6813) knots 0 0 0 1 2 2 2
  spline S179 degree 2 poles (-16.4672, 76.6813) (-16.4672, 76.5134) (-16.5215, 76.1626) (-16.566, 76.0119) knots 0 0 0 1 2 2 2
  line L195 (-16.566, 76.0119) -> (-16.9661, 76.0119)
  line L196 (-16.9661, 76.0119) -> (-16.9661, 76.0317)
  line L197 (-17.9517, 77.3235) -> (-19.2089, 77.3235)
  spline S180 degree 2 poles (-19.2089, 77.3235) (-19.2781, 77.1803) (-19.3373, 76.9382) (-19.3373, 76.8172) knots 0 0 0 1 2 2 2
  spline S181 degree 2 poles (-19.3373, 76.8172) (-19.3373, 76.5257) (-18.9076, 76.1898) (-18.5049, 76.1898) knots 0 0 0 1 2 2 2
  spline S182 degree 2 poles (-18.5049, 76.1898) (-18.1246, 76.1898) (-17.7269, 76.4442) (-17.7269, 76.7307) knots 0 0 0 1 2 2 2
  spline S183 degree 2 poles (-17.7269, 76.7307) (-17.7269, 76.8814) (-17.8454, 77.1975) (-17.9517, 77.3235) knots 0 0 0 1 2 2 2
  line L198 (-17.3317, 80.3172) -> (-20.0191, 80.3172)
  line L199 (-20.0191, 80.3172) -> (-20.0191, 79.2946)
  line L200 (-20.0191, 79.2946) -> (-20.3797, 79.2946)
  line L201 (-20.3797, 79.2946) -> (-20.3797, 81.7448)
  line L202 (-20.3797, 81.7448) -> (-20.0191, 81.7448)
  line L203 (-20.0191, 81.7448) -> (-20.0191, 80.7223)
  line L204 (-20.0191, 80.7223) -> (-17.3317, 80.7223)
  line L205 (-17.3317, 80.7223) -> (-17.3317, 80.3172)
  spline S184 degree 2 poles (-18.4753, 83.9036) (-17.8973, 83.9036) (-17.2675, 83.3479) (-17.2675, 82.8835) knots 0 0 0 1 2 2 2
  spline S185 degree 2 poles (-17.2675, 82.8835) (-17.2675, 82.4068) (-17.9171, 81.8609) (-18.4753, 81.8609) knots 0 0 0 1 2 2 2
  spline S186 degree 2 poles (-18.4753, 81.8609) (-19.0483, 81.8609) (-19.6831, 82.4241) (-19.6831, 82.8835) knots 0 0 0 1 2 2 2
  spline S187 degree 2 poles (-19.6831, 82.8835) (-19.6831, 83.3479) (-19.0508, 83.9036) (-18.4753, 83.9036) knots 0 0 0 1 2 2 2
  spline S188 degree 2 poles (-18.4753, 83.506) (-18.9199, 83.506) (-19.3522, 83.1824) (-19.3522, 82.8835) knots 0 0 0 1 2 2 2
  spline S189 degree 2 poles (-19.3522, 82.8835) (-19.3522, 82.5847) (-18.9199, 82.2586) (-18.4753, 82.2586) knots 0 0 0 1 2 2 2
  spline S190 degree 2 poles (-18.4753, 82.2586) (-18.043, 82.2586) (-17.5984, 82.5847) (-17.5984, 82.8835) knots 0 0 0 1 2 2 2
  spline S191 degree 2 poles (-17.5984, 82.8835) (-17.5984, 83.1799) (-18.0356, 83.506) (-18.4753, 83.506) knots 0 0 0 1 2 2 2
  spline S192 degree 2 poles (-18.4753, 86.1785) (-17.8973, 86.1785) (-17.2675, 85.6228) (-17.2675, 85.1584) knots 0 0 0 1 2 2 2
  spline S193 degree 2 poles (-17.2675, 85.1584) (-17.2675, 84.6817) (-17.9171, 84.1358) (-18.4753, 84.1358) knots 0 0 0 1 2 2 2
  spline S194 degree 2 poles (-18.4753, 84.1358) (-19.0483, 84.1358) (-19.6831, 84.699) (-19.6831, 85.1584) knots 0 0 0 1 2 2 2
  spline S195 degree 2 poles (-19.6831, 85.1584) (-19.6831, 85.6228) (-19.0508, 86.1785) (-18.4753, 86.1785) knots 0 0 0 1 2 2 2
  spline S196 degree 2 poles (-18.4753, 85.7809) (-18.9199, 85.7809) (-19.3522, 85.4573) (-19.3522, 85.1584) knots 0 0 0 1 2 2 2
  spline S197 degree 2 poles (-19.3522, 85.1584) (-19.3522, 84.8595) (-18.9199, 84.5335) (-18.4753, 84.5335) knots 0 0 0 1 2 2 2
  spline S198 degree 2 poles (-18.4753, 84.5335) (-18.043, 84.5335) (-17.5984, 84.8595) (-17.5984, 85.1584) knots 0 0 0 1 2 2 2
  spline S199 degree 2 poles (-17.5984, 85.1584) (-17.5984, 85.4548) (-18.0356, 85.7809) (-18.4753, 85.7809) knots 0 0 0 1 2 2 2
  line L206 (-17.3317, 86.9665) -> (-17.3317, 86.5811)
  line L207 (-17.3317, 86.5811) -> (-20.5155, 86.5811)
  line L208 (-20.5155, 86.5811) -> (-20.5155, 86.9665)
  line L209 (-20.5155, 86.9665) -> (-17.3317, 86.9665)
  point P0 (0, 0)
  constraints: 2 other
extrude "Extrusion2" cut sketch "Sketch2" against normal blind 0.254
body "Solid1"
